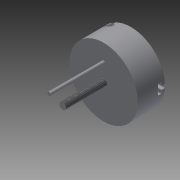
# Autodesk Inventor part: Body
Saved by Autodesk Inventor 2015 (Build 190159000, 159)
## iProperties
Created: 2016-04-14
Part Number: Body
Material: Generic
Document SubType Name: Modeling
Designer: Diogo Figueiredo
Density: 1 g/cm^3
Appearance: Default
Author: Diogo Figueiredo
Autodesk Inventor part; units mm, degrees
ref_plane "YZ Plane" through (0, 0, 0) normal (1, 0, 0) x (0, 1, 0)
ref_plane "XZ Plane" through (0, 0, 0) normal (0, 1, 0) x (-1, 0, 0)
ref_plane "XY Plane" through (0, 0, 0) normal (0, 0, 1) x (1, 0, 0)
sketch "Sketch1" plane through (0, 0, 0) normal (0, 1, 0) x (-1, 0, 0)
  circle A0 centre (0, 0) radius 50
  dimension "d0" = 100
  constraints: 1 centre point, 1 coincident
  measures "d0" diameter of A0
extrude "Extrusion1" add sketch "Sketch1" along normal blind 40
sketch "Sketch6" plane through (0, 0, 0) normal (0, -1, 0) x (1, 0, 0)
  circle A0 centre (0, 0) radius 5
  dimension "d36" = 10
  constraints: 1 centre point, 1 coincident
  measures "d36" diameter of A0
extrude "Extrusion6" add sketch "Sketch6" along normal blind 60
thread "Thread1" size "M10x1.5" class "6g" standard "ANSI Metric M Profile" full length
sketch "Sketch7" plane through (0, 40, 0) normal (0, 1, 0) x (1, 0, 0)
  line L0 (0, 0) -> (0, 50)
  circle A0 centre (0, 0) radius 5 projected
  line L1 (-27.5, -47.6314) -> (-29.6651, -46.3814)
  line L2 (-29.6651, -46.3814) -> (-26.6651, -41.1852)
  line L3 (-22.3349, -43.6852) -> (-25.3349, -48.8814)
  line L4 (-25.3349, -48.8814) -> (-27.5, -47.6314)
  line L5 (-22.3349, -43.6852) -> (-26.6651, -41.1852)
  line L6 (-27.5, 47.6314) -> (-25.3349, 48.8814)
  line L7 (-25.3349, 48.8814) -> (-22.3349, 43.6852)
  line L8 (-22.3349, 43.6852) -> (-26.6651, 41.1852)
  line L9 (-26.6651, 41.1852) -> (-29.6651, 46.3814)
  line L10 (-29.6651, 46.3814) -> (-27.5, 47.6314)
  line L11 (55, 0) -> (55, 2.5)
  line L12 (55, 2.5) -> (49, 2.5)
  line L13 (49, 2.5) -> (49, -2.5)
  line L14 (49, -2.5) -> (55, -2.5)
  line L15 (55, -2.5) -> (55, 0)
  dimension "d52" = 5
  dimension "d55" = 6
  dimension "d58" = 2.5
  dimension "d60" = 5
  constraints: 32 end point, 10 perpendicular, 3 point on line, 1 vertical
  measures "d52" distance of L2.end L3.start
  measures "d55" distance of L6.end L7.end
  measures "d58" distance of L11.start L11.end
  measures "d60" distance of L12.end L13.end
extrude "Extrusion7" cut sketch "Sketch7" against normal blind 5 contours L1 L2 L5 L3 L4 | L6 L7 L8 L9 L10 | L15 L14 L13 L12 L11
sketch "Sketch8" plane through (-22.3349, 35, -43.6852) normal (-0.5, 0, -0.866) x (-0.866, 0, 0.5)
  line L0 (0, 5) -> (5, 5)
  line L1 (5, 5) -> (5, 0)
  line L2 (5, 5) -> (5, 0) projected
  line L3 (5, 0) -> (10, 0)
  line L4 (10, 0) -> (10, -5)
  line L5 (10, -5) -> (-5, -5)
  line L6 (-5, -5) -> (-5, 0)
  line L7 (-5, 0) -> (0, 0)
  line L8 (0, 0) -> (0, 5)
  line L9 (0, 5) -> (0, 0) projected
  point P0 (2.5, -35)
  dimension "d63" = 5
  dimension "d64" = 5
  dimension "d65" = 15
  constraints: 16 end point, 5 perpendicular, 2 collinear, 1 horizontal, 1 point on line
  measures "d63" distance of L1.end L3.end
  measures "d64" distance of L3.end L4.end
  measures "d65" distance of L4.end L5.end
extrude "Extrusion8" cut sketch "Sketch8" along normal mid plane 60
sketch "Sketch9" plane through (49, 40, 2.5) normal (1, 0, 0) x (0, 0, -1)
  line L0 (5, 0) -> (0, 0)
  line L1 (0, 0) -> (5, 0) projected
  line L2 (0, 0) -> (0, -5)
  line L3 (0, -5) -> (0, 0) projected
  line L4 (0, -5) -> (-5, -5)
  line L5 (-5, -5) -> (-5, -10)
  line L6 (-5, -10) -> (10, -10)
  line L7 (10, -10) -> (10, -5)
  line L8 (10, -5) -> (5, -5)
  line L9 (5, -5) -> (5, 0)
  line L10 (5, 0) -> (5, -5) projected
  point P0 (2.5, -40)
  dimension "d68" = 5
  dimension "d69" = 5
  dimension "d70" = 15
  constraints: 16 end point, 4 perpendicular, 3 collinear, 2 point on line
  measures "d68" distance of L2.end L4.end
  measures "d69" distance of L4.end L5.end
  measures "d70" distance of L5.end L6.end
extrude "Extrusion9" cut sketch "Sketch9" along normal mid plane 60
sketch "Sketch10" plane through (-26.6651, 35, 41.1852) normal (-0.5, 0, 0.866) x (0.866, 0, 0.5)
  line L0 (5, 5) -> (0, 5)
  line L1 (0, 5) -> (5, 5) projected
  line L2 (0, 5) -> (0, 0)
  line L3 (0, 0) -> (0, 5) projected
  line L4 (0, 0) -> (-5, 0)
  line L5 (-10.2045, 0) -> (-36.5614, 0) projected
  line L6 (-5, 0) -> (-5, -5)
  line L7 (-5, -5) -> (10, -5)
  line L8 (10, -5) -> (10, 0)
  line L9 (10, 0) -> (5, 0)
  line L10 (5, 0) -> (5, 5)
  point P0 (2.5, -35)
  dimension "d73" = 5
  dimension "d74" = 5
  dimension "d75" = 15
  constraints: 16 end point, 4 perpendicular, 3 point on line, 2 collinear
  measures "d73" distance of L2.end L4.end
  measures "d74" distance of L4.end L6.end
  measures "d75" distance of L6.end L7.end
extrude "Extrusion10" cut sketch "Sketch10" along normal mid plane 60
sketch "Sketch11" plane through (0, 0, 0) normal (0, -1, 0) x (1, 0, 0)
  circle A0 centre (0, 25) radius 2.5
  point P0 (0, 0)
  dimension "d82" = 5
  constraints: 1 centre point
  measures "d82" diameter of A0
extrude "Extrusion11" add sketch "Sketch11" along normal blind 80
body "Solid1"
